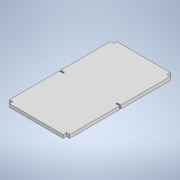
# Autodesk Inventor part: Verbinder_t80
Saved by Autodesk Inventor 2022.2 (Build 262287010, 287A)
## iProperties
Created: 2023-12-11
Part Number: Verbinder_t80
Material: Generisch
Document SubType Name: Modeling
Designer: ppovolni
Density: 1 g/cm^3
Appearance: Vorgabe
Author: ppovolni
Autodesk Inventor part; units mm, degrees
ref_plane "YZ Plane" through (0, 0, 0) normal (1, 0, 0) x (0, 1, 0)
ref_plane "XZ Plane" through (0, 0, 0) normal (0, 1, 0) x (-1, 0, 0)
ref_plane "XY Plane" through (0, 0, 0) normal (0, 0, 1) x (1, 0, 0)
sketch "Skizze1" plane through (0, 0, 0) normal (0, 1, 0) x (-1, 0, 0)
  line L0 (45, -75) -> (-45, -75)
  line L1 (-45, -75) -> (-45, 75)
  line L2 (-45, 75) -> (45, 75)
  line L3 (45, 75) -> (45, -75)
  line L4 (45, -75) -> (-45, 75) construction
  line L5 (45, 75) -> (-45, -75) construction
  line L6 (40, -75) -> (-40, -75)
  line L7 (-40, -75) -> (-40, -80)
  line L8 (-40, -80) -> (40, -80)
  line L9 (40, -80) -> (40, -75)
  line L10 (40, 75) -> (-40, 75)
  line L11 (-40, 75) -> (-40, 80)
  line L12 (-40, 80) -> (40, 80)
  line L13 (40, 80) -> (40, 75)
  line L14 (45, -1) -> (40, -1)
  line L15 (45, 1) -> (40, 1)
  line L16 (-45, -1) -> (-40, -1)
  line L17 (-45, 1) -> (-40, 1)
  arc A0 (40, 1) -> (40, -1) centre (40, 0) ccw
  arc A1 (-40, -1) -> (-40, 1) centre (-40, 0) ccw
  point P0 (0, 0)
  point P1 (0, 0)
  point P2 (40, -77.5)
  point P3 (0, 0)
  dimension "d0" = 150
  dimension "d1" = 5
  dimension "d2" = 5
  dimension "d3" = 5
  dimension "d4" = 80
  dimension "d5" = 2
  dimension "d6" = 5
  dimension "d7" = 1
  constraints: 36 end point, 7 horizontal, 6 parallel, 6 point on line, 4 collinear, 4 equal length, 4 point on circle, 3 midpoint, 3 perpendicular, 2 centre point, 2 tangent, 1 coincident
  measures "d0" distance of L2.end L0.start
  measures "d1" distance between parallel lines of L1 L7
  measures "d2" distance from line of L3 point (40, -77.5)
  measures "d3" distance of L6.end L7.end
  measures "d4" distance of L7.end L8.end
  measures "d5" distance between parallel lines of L15 L14
  measures "d6" distance of L14.start L14.end
  measures "d7" distance from line of L15 point (0, 0)
extrude "Extrusion1" add sketch "Skizze1" along normal blind 5 contours L0 L1 L16 A1 L17 L2 L3 L15 A0 L14 | L9 L8 L7 L0 | L2 L11 L12 L13
equation "\"d4\" = t"
equation "\"t\" = 80"
